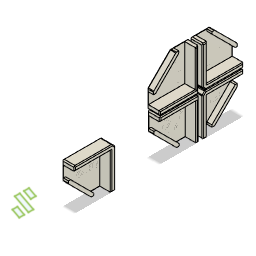
extrusion door corners v3 (Autodesk Fusion 360 design; units mm, degrees)
Autodesk Fusion 360 part; units mm, degrees
note: some values were not read from the file. Chosen so that the rebuilt part matches the saved one: which pieces of a blend or face edit are solid.
sketch "Sketch1" plane through (0, 0, 0) normal (0, 1, 0) x (1, 0, 0)
  line L0 (2, 2) -> (8, 2)
  line L1 (8, 2) -> (8, 8)
  line L2 (8, 8) -> (2, 8)
  line L3 (2, 8) -> (2, 2)
  line L4 (3.7738, 2) -> (6.1738, 2)
  line L5 (6.1738, 2) -> (6.1738, 6)
  line L6 (6.1738, 6) -> (3.7738, 6)
  line L7 (3.7738, 6) -> (3.7738, 2)
  dimension "d1" = 6
  dimension "d2" = 6
  dimension "d3" = 2.4
  dimension "d4" = 4
  constraint horizontal L0
  constraint vertical L1
  constraint horizontal L2
  constraint vertical L3
  constraint horizontal L4
  constraint vertical L5
  constraint horizontal L6
  constraint vertical L7
  constraint coincident L0 L4.start
  measures "d1" distance of L0.start L0.end
  measures "d2" distance of L0.start L2.end
  measures "d3" distance of L4.start L4.end
  measures "d4" distance of L4.start L6.end
sketch "Sketch2" plane through (0, 0, 0) normal (1, 0, 0) x (0, 0, -1)
  line L0 (-1.5, 1) -> (-73.5, 1)
  line L1 (-73.5, 1) -> (-73.5, 73)
  line L2 (-73.5, 73) -> (-1.5, 73)
  line L3 (-1.5, 73) -> (-1.5, 1)
  dimension "d20" = 72
  dimension "d21" = 72
  constraint horizontal L0
  constraint vertical L1
  constraint horizontal L2
  constraint vertical L3
  measures "d20" distance of L0.start L0.end
  measures "d21" distance of L0.start L2.end
extrude "Extrude2" add sketch "Sketch2" along normal blind 2 makes body 1
sketch "Sketch3" plane through (2, 0, 0) normal (1, 0, 0) x (0, 0, -1)
  line L0 (-1.5, 73) -> (-73.5, 73)
  line L1 (-73.5, 73) -> (-73.5, 1)
  line L2 (-73.5, 1) -> (-1.5, 1)
  line L3 (-1.5, 1) -> (-1.5, 73)
  line L4 (-1.5, 1) -> (-73.5, 1)
  line L5 (-73.5, 1) -> (-73.5, 8.8)
  line L6 (-73.5, 8.8) -> (-1.5, 8.8)
  line L7 (-1.5, 8.8) -> (-1.5, 1)
  line L8 (-1.5, 8.8) -> (-9.3, 8.8)
  line L9 (-9.3, 8.8) -> (-9.3, 73)
  line L10 (-9.3, 73) -> (-1.5, 73)
  line L11 (-1.5, 73) -> (-1.5, 8.8)
  dimension "d24" = 7.8
  dimension "d25" = 7.8
  constraint horizontal L4
  constraint vertical L5
  constraint horizontal L6
  constraint vertical L7
  constraint coincident L2.end L3.start
  constraint horizontal L8
  constraint vertical L9
  constraint horizontal L10
  constraint vertical L11
  measures "d24" distance of L2.end L6.end
  measures "d25" distance of L6.end L8.end
extrude "Extrude3" add sketch "Sketch3" along normal blind 20 contours L1 L2 L3 L4 L5 L6 L7 L8 bodies 1
sketch "Sketch4" plane through (2, 0, 0) normal (1, 0, 0) x (0, 0, -1)
  line L0 (-73.5, 8.8) -> (-1.5, 8.8)
  line L1 (-1.5, 8.8) -> (-1.5, 73)
  line L2 (-1.5, 73) -> (-73.5, 73)
  line L3 (-73.5, 73) -> (-73.5, 8.8)
  line L4 (-1.5, 8.8) -> (-9.3, 8.8)
  line L5 (-9.3, 8.8) -> (-9.3, 73)
  line L6 (-9.3, 73) -> (-1.5, 73)
  line L7 (-1.5, 73) -> (-1.5, 8.8)
  dimension "d28" = 7.8
  constraint horizontal L4
  constraint vertical L5
  constraint horizontal L6
  constraint vertical L7
  constraint coincident L0.end L1.start
  measures "d28" distance of L0.end L4.end
extrude "Extrude4" add sketch "Sketch4" along normal blind 7.8 contours L0 L1 L2 L4 L5 L6 L7 bodies 1
sketch "Sketch5" plane through (2, 0, 0) normal (1, 0, 0) x (0, 0, -1)
  line L0 (-9.3, 8.8) -> (-9.3, 73)
  line L1 (-9.3, 73) -> (-73.5, 73)
  line L2 (-73.5, 73) -> (-73.5, 8.8)
  line L3 (-73.5, 8.8) -> (-9.3, 8.8)
  line L4 (-73.5, 73) -> (-28.828, 73)
  line L5 (-28.828, 73) -> (-28.828, 28.328)
  line L6 (-28.828, 28.328) -> (-73.5, 28.328)
  line L7 (-73.5, 28.328) -> (-73.5, 73)
  dimension "d31" = 44.672
  dimension "d32" = 44.672
  constraint horizontal L4
  constraint vertical L5
  constraint horizontal L6
  constraint vertical L7
  constraint coincident L1.end L2.start
  measures "d31" distance of L1.end L4.end
  measures "d32" distance of L1.end L6.end
extrude "Extrude5" add sketch "Sketch5" along normal blind 9 contours L1 L2 L4 L5 L6 L7 bodies 1
extrude "Extrude6" add 1 faces at (9.8, 51.6, 6.7) along direction (1, 0, 0) blind 12 on bodies 1 bodies 1
extrude "Extrude7" add 1 faces at (21.8, 51.6, 6.7) along direction (1, 0, 0) blind 0.2 on bodies 1 bodies 1
chamfer "Chamfer6" distance 40 angle 45 1 edges at (5.5, 73, 73.5) on bodies 1
chamfer "Chamfer9" distance 41 angle 45 1 edges at (6.5, 28.328, 28.828) on bodies 1
chamfer "Chamfer12" distance 1.5 angle 45 1 faces at (0, 35.6667, 36.1667) on bodies 1
chamfer "Chamfer13" distance 1.5 angle 45 1 faces at (22, 3.6, 28.1) on bodies 1
fillet "Fillet4" radius 2 4 edges at (11, 1, 73.5) (6.25, 73, 33.5) (6.25, 33, 73.5) (11, 73, 1.5) on bodies 1
chamfer "Chamfer14" distance 5 angle 45 1 edges at (11, 1, 1.5) on bodies 1
chamfer "Chamfer15" distance 1.5 angle 45 2 edges at (0, 3.5, 4) (22, 3.5, 4) on bodies 1
fillet "Fillet5" radius 2 2 edges at (11, 1, 6.5) (11, 6, 1.5) on bodies 1
sketch "Sketch6" plane through (0, 0, 0) normal (1, 0, 0) x (0, 0, -1)
  line L0 (37.7693, -15.5046) -> (28.9904, -15.5046)
  line L1 (28.9904, -15.5046) -> (40.9998, -33.7714)
  line L2 (40.9998, -33.7714) -> (49.7787, -33.7714)
  line L3 (49.7787, -33.7714) -> (37.7693, -15.5046)
  line L4 (45.6089, -52.0171) -> (21.5926, -15.4781)
  line L5 (21.5926, -15.4781) -> (12.8138, -15.4781)
  line L6 (12.8138, -15.4781) -> (36.8327, -52.0171)
  line L7 (36.8327, -52.0171) -> (45.6089, -52.0171)
  line L8 (20.6507, -52.0171) -> (29.4296, -52.0171)
  line L9 (29.4296, -52.0171) -> (17.4228, -33.7503)
  line L10 (17.4228, -33.7503) -> (8.6439, -33.7503)
  line L11 (8.6439, -33.7503) -> (20.6507, -52.0171)
copy_body "CopyPasteBodies1" bodies 1 makes body 2
move_body "Move1" bodies 2 to x (1, 0, 0) y (0, 1, 0) z (0, 0, 1) at (0, 0, 155)
mirror "Mirror1" about plane through (0, 0, 0) normal (0, 0, 1) of bodies 2 makes body 3
mirror "Mirror2" about plane through (0, 0, 0) normal (0, 1, 0) of bodies 3 makes body 4
mirror "Mirror3" about plane through (0, 0, 0) normal (0, 1, 0) of bodies 1 makes body 5
move_body "Move2" bodies 1 to x (1, 0, 0) y (0, 1, 0) z (0, 0, 1) at (0, 0, -320)
move_body "Move3" bodies 4 to x (1, 0, 0) y (0, 1, 0) z (0, 0, 1) at (0, 150, 0)
move_body "Move4" bodies 5 to x (1, 0, 0) y (0, 1, 0) z (0, 0, 1) at (0, 150, -320)
sketch "Sketch7" plane through (0, 0, 0) normal (-1, 0, 0) x (0, 0, 1)
  line L0 (-162.1213, 2.5) -> (-158, 6.6213)
  line L1 (-158, 6.6213) -> (-158, 71.5)
  line L2 (-158, 71.5) -> (-187.8787, 71.5)
  line L3 (-187.8787, 71.5) -> (-227, 32.3787)
  line L4 (-227, 32.3787) -> (-227, 2.5)
  line L5 (-227, 2.5) -> (-162.1213, 2.5)
  line L6 (-196.3905, 49.0459) -> (-188.4895, 49.0459)
  line L7 (-188.4895, 49.0459) -> (-199.298, 32.6057)
  line L8 (-199.298, 32.6057) -> (-207.199, 32.6057)
  line L9 (-207.199, 32.6057) -> (-196.3905, 49.0459)
  line L10 (-203.4462, 16.1846) -> (-181.8316, 49.0697)
  line L11 (-181.8316, 49.0697) -> (-173.9306, 49.0697)
  line L12 (-173.9306, 49.0697) -> (-195.5476, 16.1846)
  line L13 (-195.5476, 16.1846) -> (-203.4462, 16.1846)
  line L14 (-180.9838, 16.1846) -> (-188.8848, 16.1846)
  line L15 (-188.8848, 16.1846) -> (-178.0787, 32.6248)
  line L16 (-178.0787, 32.6248) -> (-170.1777, 32.6248)
  line L17 (-170.1777, 32.6248) -> (-180.9838, 16.1846)
extrude "Extrude8" cut sketch "Sketch7" against normal blind 0.7 contours L6 L7 L8 L9 | L10 L11 L12 L13 | L14 L15 L16 L17 bodies 3
sketch "Sketch8" plane through (0, 0, 0) normal (-1, 0, 0) x (0, 0, 1)
  line L0 (-317, 6.6213) -> (-312.8787, 2.5)
  line L1 (-312.8787, 2.5) -> (-248, 2.5)
  line L2 (-248, 2.5) -> (-248, 32.3787)
  line L3 (-248, 32.3787) -> (-287.1213, 71.5)
  line L4 (-287.1213, 71.5) -> (-317, 71.5)
  line L5 (-317, 71.5) -> (-317, 6.6213)
  line L6 (-296.3905, 49.0459) -> (-288.4895, 49.0459)
  line L7 (-288.4895, 49.0459) -> (-299.298, 32.6057)
  line L8 (-299.298, 32.6057) -> (-307.199, 32.6057)
  line L9 (-307.199, 32.6057) -> (-296.3905, 49.0459)
  line L10 (-303.4462, 16.1846) -> (-281.8316, 49.0697)
  line L11 (-281.8316, 49.0697) -> (-273.9306, 49.0697)
  line L12 (-273.9306, 49.0697) -> (-295.5476, 16.1846)
  line L13 (-295.5476, 16.1846) -> (-303.4462, 16.1846)
  line L14 (-280.9838, 16.1846) -> (-288.8848, 16.1846)
  line L15 (-288.8848, 16.1846) -> (-278.0787, 32.6248)
  line L16 (-278.0787, 32.6248) -> (-270.1777, 32.6248)
  line L17 (-270.1777, 32.6248) -> (-280.9838, 16.1846)
extrude "Extrude9" cut sketch "Sketch8" against normal blind 0.7 contours L6 L7 L8 L9 | L10 L11 L12 L13 | L14 L15 L16 L17 bodies 1
sketch "Sketch9" plane through (0, 0, 0) normal (-1, 0, 0) x (0, 0, 1)
  line L0 (-158, 143.3787) -> (-162.1213, 147.5)
  line L1 (-162.1213, 147.5) -> (-227, 147.5)
  line L2 (-227, 147.5) -> (-227, 117.6213)
  line L3 (-227, 117.6213) -> (-187.8787, 78.5)
  line L4 (-187.8787, 78.5) -> (-158, 78.5)
  line L5 (-158, 78.5) -> (-158, 143.3787)
  line L6 (-164.2409, 106.1512) -> (-169.8403, 106.1512)
  line L7 (-169.8403, 106.1512) -> (-176.0067, 124.5441)
  line L8 (-176.0067, 124.5441) -> (-176.1485, 124.5441)
  line L9 (-176.1485, 124.5441) -> (-182.3149, 106.1512)
  line L10 (-182.3149, 106.1512) -> (-187.7725, 106.1512)
  line L11 (-187.7725, 106.1512) -> (-179.2671, 129.1512)
  line L12 (-179.2671, 129.1512) -> (-172.4983, 129.1512)
  line L13 (-172.4983, 129.1512) -> (-164.2409, 106.1512)
  spline S0 degree 2 poles (-189.828, 123.9062) (-189.828, 121.9925) (-190.8912, 120.5749) knots 0 0 0 1 1 1
  spline S1 degree 2 poles (-190.8912, 120.5749) (-191.9544, 119.1573) (-193.6554, 118.4131) knots 0 0 0 1 1 1
  spline S2 degree 2 poles (-193.6554, 118.4131) (-195.0021, 117.8107) (-196.8095, 117.2082) knots 0 0 0 1 1 1
  spline S3 degree 2 poles (-196.8095, 117.2082) (-198.6169, 116.6057) (-199.6092, 115.9324) knots 0 0 0 1 1 1
  spline S4 degree 2 poles (-199.6092, 115.9324) (-200.6015, 115.259) (-200.6015, 114.3376) knots 0 0 0 1 1 1
  line L14 (-200.6015, 114.3376) -> (-200.6015, 111.3962)
  spline S5 degree 2 poles (-200.6015, 111.3962) (-200.6015, 110.2976) (-199.7155, 109.9432) knots 0 0 0 1 1 1
  spline S6 degree 2 poles (-199.7155, 109.9432) (-198.7587, 109.5533) (-196.7386, 109.5533) knots 0 0 0 1 1 1
  spline S7 degree 2 poles (-196.7386, 109.5533) (-194.2933, 109.5533) (-190.2887, 110.4393) knots 0 0 0 1 1 1
  line L15 (-190.2887, 110.4393) -> (-190.2887, 106.541)
  spline S8 degree 2 poles (-190.2887, 106.541) (-193.8326, 105.7968) (-197.6955, 105.7968) knots 0 0 0 1 1 1
  spline S9 degree 2 poles (-197.6955, 105.7968) (-201.8773, 105.7968) (-203.9151, 107.0726) knots 0 0 0 1 1 1
  spline S10 degree 2 poles (-203.9151, 107.0726) (-205.9528, 108.3484) (-205.9528, 111.3253) knots 0 0 0 1 1 1
  line L16 (-205.9528, 111.3253) -> (-205.9528, 114.5148)
  spline S11 degree 2 poles (-205.9528, 114.5148) (-205.9528, 116.3222) (-204.8719, 117.6512) knots 0 0 0 1 1 1
  spline S12 degree 2 poles (-204.8719, 117.6512) (-203.791, 118.9801) (-202.0899, 119.6535) knots 0 0 0 1 1 1
  spline S13 degree 2 poles (-202.0899, 119.6535) (-200.4952, 120.3268) (-198.8295, 120.8584) knots 0 0 0 1 1 1
  spline S14 degree 2 poles (-198.8295, 120.8584) (-197.0222, 121.4963) (-195.9767, 122.276) knots 0 0 0 1 1 1
  spline S15 degree 2 poles (-195.9767, 122.276) (-194.9312, 123.0556) (-194.9312, 124.1188) knots 0 0 0 1 1 1
  line L17 (-194.9312, 124.1188) -> (-194.9312, 125.2883)
  line L18 (-194.9312, 125.2883) -> (-205.9883, 125.2883)
  line L19 (-205.9883, 125.2883) -> (-205.9883, 129.1512)
  line L20 (-205.9883, 129.1512) -> (-189.828, 129.1512)
  line L21 (-189.828, 129.1512) -> (-189.828, 123.9062)
extrude "Extrude10" cut sketch "Sketch9" against normal blind 0.7 contours L6 L7 L8 L9 L10 L11 L12 L13 | S0 S1 S2 S3 S4 L14 S5 S6 S7 L15 S8 S9 S10 L16 S11 S12 S13 S14 S15 L17 L18 L19 L20 L21 bodies 4
sketch "Sketch10" plane through (0, 0, 0) normal (-1, 0, 0) x (0, 0, 1)
  line L0 (-312.8787, 147.5) -> (-317, 143.3787)
  line L1 (-317, 143.3787) -> (-317, 78.5)
  line L2 (-317, 78.5) -> (-287.1213, 78.5)
  line L3 (-287.1213, 78.5) -> (-248, 117.6213)
  line L4 (-248, 117.6213) -> (-248, 147.5)
  line L5 (-248, 147.5) -> (-312.8787, 147.5)
  line L6 (-168.6342, 139.35) -> (-167.4416, 139.35)
  line L7 (-167.4416, 139.35) -> (-167.4416, 138.2544)
  line L8 (-167.4416, 138.2544) -> (-168.8561, 138.2544)
  line L9 (-168.8561, 138.2544) -> (-169.1612, 136.8122)
  line L10 (-169.1612, 136.8122) -> (-167.4416, 136.8122)
  line L11 (-167.4416, 136.8122) -> (-167.4416, 135.7028)
  line L12 (-167.4416, 135.7028) -> (-169.3831, 135.7028)
  line L13 (-169.3831, 135.7028) -> (-169.8962, 133.1651)
  line L14 (-169.8962, 133.1651) -> (-171.0888, 133.1651)
  line L15 (-171.0888, 133.1651) -> (-170.5757, 135.7028)
  line L16 (-170.5757, 135.7028) -> (-171.4632, 135.7028)
  line L17 (-171.4632, 135.7028) -> (-171.9763, 133.1651)
  line L18 (-171.9763, 133.1651) -> (-173.1689, 133.1651)
  line L19 (-173.1689, 133.1651) -> (-172.6558, 135.7028)
  line L20 (-172.6558, 135.7028) -> (-173.8207, 135.7028)
  line L21 (-173.8207, 135.7028) -> (-173.8207, 136.8122)
  line L22 (-173.8207, 136.8122) -> (-172.4201, 136.8122)
  line L23 (-172.4201, 136.8122) -> (-172.1288, 138.2544)
  line L24 (-172.1288, 138.2544) -> (-173.8207, 138.2544)
  line L25 (-173.8207, 138.2544) -> (-173.8207, 139.35)
  line L26 (-173.8207, 139.35) -> (-171.907, 139.35)
  line L27 (-171.907, 139.35) -> (-171.3661, 142.0264)
  line L28 (-171.3661, 142.0264) -> (-170.1735, 142.0264)
  line L29 (-170.1735, 142.0264) -> (-170.7144, 139.35)
  line L30 (-170.7144, 139.35) -> (-169.8268, 139.35)
  line L31 (-169.8268, 139.35) -> (-169.286, 142.0264)
  line L32 (-169.286, 142.0264) -> (-168.0934, 142.0264)
  line L33 (-168.0934, 142.0264) -> (-168.6342, 139.35)
  line L34 (-170.9362, 138.2544) -> (-171.2413, 136.8122)
  line L35 (-171.2413, 136.8122) -> (-170.3399, 136.8122)
  line L36 (-170.3399, 136.8122) -> (-170.0487, 138.2544)
  line L37 (-170.0487, 138.2544) -> (-170.9362, 138.2544)
  line L38 (-178.286, 135.1481) -> (-175.8315, 136.5071)
  line L39 (-175.8315, 136.5071) -> (-175.8315, 134.8014)
  line L40 (-175.8315, 134.8014) -> (-178.6743, 133.0264)
  line L41 (-178.6743, 133.0264) -> (-180.3107, 133.0264)
  line L42 (-180.3107, 133.0264) -> (-180.3107, 142.0264)
  line L43 (-180.3107, 142.0264) -> (-178.286, 142.0264)
  line L44 (-178.286, 142.0264) -> (-178.286, 135.1481)
  line L45 (-186.3291, 135.1481) -> (-183.8746, 136.5071)
  line L46 (-183.8746, 136.5071) -> (-183.8746, 134.8014)
  line L47 (-183.8746, 134.8014) -> (-186.7174, 133.0264)
  line L48 (-186.7174, 133.0264) -> (-188.3538, 133.0264)
  line L49 (-188.3538, 133.0264) -> (-188.3538, 142.0264)
  line L50 (-188.3538, 142.0264) -> (-186.3291, 142.0264)
  line L51 (-186.3291, 142.0264) -> (-186.3291, 135.1481)
  line L52 (-195.2598, 140.2097) -> (-191.0996, 140.2097)
  line L53 (-191.0996, 140.2097) -> (-191.0996, 138.615)
  line L54 (-191.0996, 138.615) -> (-194.8022, 133.0264)
  line L55 (-194.8022, 133.0264) -> (-197.0903, 133.0264)
  line L56 (-197.0903, 133.0264) -> (-197.0903, 138.7537)
  line L57 (-197.0903, 138.7537) -> (-198.061, 138.7537)
  line L58 (-198.061, 138.7537) -> (-198.061, 140.2097)
  line L59 (-198.061, 140.2097) -> (-197.0903, 140.2097)
  line L60 (-197.0903, 140.2097) -> (-197.0903, 142.0264)
  line L61 (-197.0903, 142.0264) -> (-195.2598, 142.0264)
  line L62 (-195.2598, 142.0264) -> (-195.2598, 140.2097)
  line L63 (-195.2598, 138.7537) -> (-195.2598, 134.9401)
  line L64 (-195.2598, 134.9401) -> (-192.833, 138.7537)
  line L65 (-192.833, 138.7537) -> (-195.2598, 138.7537)
  spline S0 degree 2 poles (-202.457, 142.1651) (-201.2922, 142.1651) (-199.4339, 141.957) knots 0 0 0 1 1 1
  line L66 (-199.4339, 141.957) -> (-199.4339, 140.3484)
  line L67 (-199.4339, 140.3484) -> (-199.8777, 140.4316)
  spline S1 degree 2 poles (-199.8777, 140.4316) (-200.1412, 140.4871) (-200.1689, 140.501) knots 0 0 0 1 1 1
  line L68 (-200.1689, 140.501) -> (-200.6404, 140.5842)
  spline S2 degree 2 poles (-200.6404, 140.5842) (-200.8068, 140.6119) (-201.3476, 140.6674) knots 0 0 0 1 1 1
  spline S3 degree 2 poles (-201.3476, 140.6674) (-201.7637, 140.709) (-202.1936, 140.709) knots 0 0 0 1 1 1
  spline S4 degree 2 poles (-202.1936, 140.709) (-202.9979, 140.709) (-203.3099, 140.5148) knots 0 0 0 1 1 1
  spline S5 degree 2 poles (-203.3099, 140.5148) (-203.6219, 140.3207) (-203.6219, 139.7799) knots 0 0 0 1 1 1
  line L69 (-203.6219, 139.7799) -> (-203.6219, 138.7398)
  spline S6 degree 2 poles (-203.6219, 138.7398) (-203.6219, 138.088) (-202.2213, 138.088) knots 0 0 0 1 1 1
  line L70 (-202.2213, 138.088) -> (-200.5849, 138.088)
  line L71 (-200.5849, 138.088) -> (-200.5849, 136.7013)
  line L72 (-200.5849, 136.7013) -> (-202.2213, 136.7013)
  spline S7 degree 2 poles (-202.2213, 136.7013) (-203.303, 136.7013) (-203.303, 135.9108) knots 0 0 0 1 1 1
  line L73 (-203.303, 135.9108) -> (-203.303, 135.0372)
  spline S8 degree 2 poles (-203.303, 135.0372) (-203.303, 134.746) (-203.192, 134.5865) knots 0 0 0 1 1 1
  spline S9 degree 2 poles (-203.192, 134.5865) (-203.0811, 134.427) (-202.7968, 134.3577) knots 0 0 0 1 1 1
  spline S10 degree 2 poles (-202.7968, 134.3577) (-202.5125, 134.2883) (-201.9578, 134.2883) knots 0 0 0 1 1 1
  spline S11 degree 2 poles (-201.9578, 134.2883) (-201.1674, 134.2883) (-199.5171, 134.4547) knots 0 0 0 1 1 1
  line L74 (-199.5171, 134.4547) -> (-199.5171, 133.0125)
  spline S12 degree 2 poles (-199.5171, 133.0125) (-201.4031, 132.8877) (-202.1797, 132.8877) knots 0 0 0 1 1 1
  spline S13 degree 2 poles (-202.1797, 132.8877) (-203.8715, 132.8877) (-204.6273, 133.276) knots 0 0 0 1 1 1
  spline S14 degree 2 poles (-204.6273, 133.276) (-205.3831, 133.6643) (-205.3831, 134.6489) knots 0 0 0 1 1 1
  line L75 (-205.3831, 134.6489) -> (-205.3831, 136.1327)
  spline S15 degree 2 poles (-205.3831, 136.1327) (-205.3831, 136.5349) (-205.1404, 136.8191) knots 0 0 0 1 1 1
  spline S16 degree 2 poles (-205.1404, 136.8191) (-204.8977, 137.1034) (-204.5233, 137.2005) knots 0 0 0 1 1 1
  spline S17 degree 2 poles (-204.5233, 137.2005) (-205.7436, 137.6304) (-205.7436, 138.5456) knots 0 0 0 1 1 1
  line L76 (-205.7436, 138.5456) -> (-205.7436, 140.0156)
  spline S18 degree 2 poles (-205.7436, 140.0156) (-205.7436, 141.1666) (-204.9532, 141.6658) knots 0 0 0 1 1 1
  spline S19 degree 2 poles (-204.9532, 141.6658) (-204.1627, 142.1651) (-202.457, 142.1651) knots 0 0 0 1 1 1
  line L77 (-267.4991, 108.339) -> (-269.9028, 108.339)
  line L78 (-269.9028, 108.339) -> (-269.9028, 118.339)
  line L79 (-269.9028, 118.339) -> (-267.4991, 118.339)
  line L80 (-267.4991, 118.339) -> (-267.4991, 108.339)
  line L81 (-269.9644, 113.0385) -> (-273.7087, 108.339)
  line L82 (-273.7087, 108.339) -> (-276.5284, 108.339)
  line L83 (-276.5284, 108.339) -> (-272.7379, 112.9923)
  line L84 (-272.7379, 112.9923) -> (-276.9444, 118.339)
  line L85 (-276.9444, 118.339) -> (-274.0168, 118.339)
  line L86 (-274.0168, 118.339) -> (-269.9644, 113.0385)
  line L87 (-280.6732, 114.3328) -> (-277.0523, 108.339)
  line L88 (-277.0523, 108.339) -> (-279.7795, 108.339)
  line L89 (-279.7795, 108.339) -> (-281.8905, 112.2527)
  line L90 (-281.8905, 112.2527) -> (-283.986, 108.339)
  line L91 (-283.986, 108.339) -> (-286.7287, 108.339)
  line L92 (-286.7287, 108.339) -> (-283.0769, 114.302)
  line L93 (-283.0769, 114.302) -> (-283.0769, 118.339)
  line L94 (-283.0769, 118.339) -> (-280.6732, 118.339)
  line L95 (-280.6732, 118.339) -> (-280.6732, 114.3328)
  line L96 (-287.9305, 108.339) -> (-292.4298, 108.339)
  spline S20 degree 2 poles (-292.4298, 108.339) (-294.4329, 108.339) (-295.3265, 108.8243) knots 0 0 0 1 1 1
  spline S21 degree 2 poles (-295.3265, 108.8243) (-296.2202, 109.3097) (-296.2202, 110.4499) knots 0 0 0 1 1 1
  line L97 (-296.2202, 110.4499) -> (-296.2202, 112.2065)
  spline S22 degree 2 poles (-296.2202, 112.2065) (-296.2202, 113.0847) (-295.5962, 113.5855) knots 0 0 0 1 1 1
  spline S23 degree 2 poles (-295.5962, 113.5855) (-294.9721, 114.0863) (-293.9398, 114.225) knots 0 0 0 1 1 1
  line L98 (-293.9398, 114.225) -> (-296.8366, 118.339)
  line L99 (-296.8366, 118.339) -> (-294.0631, 118.339)
  line L100 (-294.0631, 118.339) -> (-291.4436, 114.4099)
  line L101 (-291.4436, 114.4099) -> (-290.3342, 114.4099)
  line L102 (-290.3342, 114.4099) -> (-290.3342, 118.339)
  line L103 (-290.3342, 118.339) -> (-287.9305, 118.339)
  line L104 (-287.9305, 118.339) -> (-287.9305, 108.339)
  spline S24 degree 2 poles (-292.399, 112.8228) (-293.2464, 112.8228) (-293.5546, 112.5994) knots 0 0 0 1 1 1
  spline S25 degree 2 poles (-293.5546, 112.5994) (-293.8627, 112.376) (-293.8627, 111.7288) knots 0 0 0 1 1 1
  line L105 (-293.8627, 111.7288) -> (-293.8627, 111.02)
  spline S26 degree 2 poles (-293.8627, 111.02) (-293.8627, 110.4653) (-293.5315, 110.2573) knots 0 0 0 1 1 1
  spline S27 degree 2 poles (-293.5315, 110.2573) (-293.2002, 110.0493) (-292.399, 110.0493) knots 0 0 0 1 1 1
  line L106 (-292.399, 110.0493) -> (-290.3342, 110.0493)
  line L107 (-290.3342, 110.0493) -> (-290.3342, 112.8228)
  line L108 (-290.3342, 112.8228) -> (-292.399, 112.8228)
  spline S28 degree 2 poles (-302.7379, 118.4931) (-301.9059, 118.4931) (-301.2048, 118.3852) knots 0 0 0 1 1 1
  spline S29 degree 2 poles (-301.2048, 118.3852) (-300.5037, 118.2774) (-299.7487, 118.0154) knots 0 0 0 1 1 1
  spline S30 degree 2 poles (-299.7487, 118.0154) (-298.9321, 117.7381) (-298.4698, 117.114) knots 0 0 0 1 1 1
  spline S31 degree 2 poles (-298.4698, 117.114) (-298.0076, 116.49) (-298.0076, 115.5963) knots 0 0 0 1 1 1
  line L109 (-298.0076, 115.5963) -> (-298.0076, 111.2203)
  spline S32 degree 2 poles (-298.0076, 111.2203) (-298.0076, 110.4807) (-298.3389, 109.8952) knots 0 0 0 1 1 1
  spline S33 degree 2 poles (-298.3389, 109.8952) (-298.6701, 109.3097) (-299.194, 108.9707) knots 0 0 0 1 1 1
  spline S34 degree 2 poles (-299.194, 108.9707) (-299.6563, 108.678) (-300.3342, 108.4777) knots 0 0 0 1 1 1
  spline S35 degree 2 poles (-300.3342, 108.4777) (-301.0122, 108.2774) (-301.5977, 108.2311) knots 0 0 0 1 1 1
  spline S36 degree 2 poles (-301.5977, 108.2311) (-302.137, 108.1849) (-302.7379, 108.1849) knots 0 0 0 1 1 1
  spline S37 degree 2 poles (-302.7379, 108.1849) (-303.4467, 108.1849) (-303.9706, 108.2388) knots 0 0 0 1 1 1
  spline S38 degree 2 poles (-303.9706, 108.2388) (-304.4945, 108.2928) (-305.1416, 108.4623) knots 0 0 0 1 1 1
  spline S39 degree 2 poles (-305.1416, 108.4623) (-305.8812, 108.678) (-306.3589, 108.9861) knots 0 0 0 1 1 1
  spline S40 degree 2 poles (-306.3589, 108.9861) (-306.8366, 109.2943) (-307.1601, 109.849) knots 0 0 0 1 1 1
  spline S41 degree 2 poles (-307.1601, 109.849) (-307.4991, 110.4191) (-307.4991, 111.2203) knots 0 0 0 1 1 1
  line L110 (-307.4991, 111.2203) -> (-307.4991, 115.5963)
  spline S42 degree 2 poles (-307.4991, 115.5963) (-307.4991, 116.4284) (-307.06, 117.0293) knots 0 0 0 1 1 1
  spline S43 degree 2 poles (-307.06, 117.0293) (-306.6208, 117.6302) (-305.8504, 117.9384) knots 0 0 0 1 1 1
  spline S44 degree 2 poles (-305.8504, 117.9384) (-304.4637, 118.4931) (-302.7379, 118.4931) knots 0 0 0 1 1 1
  spline S45 degree 2 poles (-302.7688, 116.7827) (-303.2772, 116.7827) (-303.6239, 116.7442) knots 0 0 0 1 1 1
  spline S46 degree 2 poles (-303.6239, 116.7442) (-303.9706, 116.7057) (-304.3404, 116.5978) knots 0 0 0 1 1 1
  spline S47 degree 2 poles (-304.3404, 116.5978) (-304.7102, 116.49) (-304.9028, 116.2357) knots 0 0 0 1 1 1
  spline S48 degree 2 poles (-304.9028, 116.2357) (-305.0954, 115.9815) (-305.0954, 115.5963) knots 0 0 0 1 1 1
  line L111 (-305.0954, 115.5963) -> (-305.0954, 111.2049)
  spline S49 degree 2 poles (-305.0954, 111.2049) (-305.0954, 110.4962) (-304.5253, 110.1957) knots 0 0 0 1 1 1
  spline S50 degree 2 poles (-304.5253, 110.1957) (-303.9552, 109.8952) (-302.7533, 109.8952) knots 0 0 0 1 1 1
  spline S51 degree 2 poles (-302.7533, 109.8952) (-301.5515, 109.8952) (-300.9814, 110.188) knots 0 0 0 1 1 1
  spline S52 degree 2 poles (-300.9814, 110.188) (-300.4113, 110.4807) (-300.4113, 111.2049) knots 0 0 0 1 1 1
  line L112 (-300.4113, 111.2049) -> (-300.4113, 115.5963)
  spline S53 degree 2 poles (-300.4113, 115.5963) (-300.4113, 115.9815) (-300.6116, 116.2357) knots 0 0 0 1 1 1
  spline S54 degree 2 poles (-300.6116, 116.2357) (-300.8119, 116.49) (-301.1971, 116.5978) knots 0 0 0 1 1 1
  spline S55 degree 2 poles (-301.1971, 116.5978) (-301.5669, 116.7057) (-301.9136, 116.7442) knots 0 0 0 1 1 1
  spline S56 degree 2 poles (-301.9136, 116.7442) (-302.2603, 116.7827) (-302.7688, 116.7827) knots 0 0 0 1 1 1
  line L113 (-269.2942, 128) -> (-271.6979, 128)
  line L114 (-271.6979, 128) -> (-271.6979, 136.2897)
  line L115 (-271.6979, 136.2897) -> (-276.6131, 136.2897)
  line L116 (-276.6131, 136.2897) -> (-276.6131, 138)
  line L117 (-276.6131, 138) -> (-269.2942, 138)
  line L118 (-269.2942, 138) -> (-269.2942, 128)
  line L119 (-280.8812, 128) -> (-283.8088, 128)
  line L120 (-283.8088, 128) -> (-287.4144, 138)
  line L121 (-287.4144, 138) -> (-284.9799, 138)
  line L122 (-284.9799, 138) -> (-284.0862, 135.3652)
  line L123 (-284.0862, 135.3652) -> (-280.4344, 135.3652)
  line L124 (-280.4344, 135.3652) -> (-279.5561, 138)
  line L125 (-279.5561, 138) -> (-277.1832, 138)
  line L126 (-277.1832, 138) -> (-280.8812, 128)
  line L127 (-283.5623, 133.7627) -> (-282.2988, 130.0031)
  line L128 (-282.2988, 130.0031) -> (-282.2372, 130.0031)
  line L129 (-282.2372, 130.0031) -> (-280.9737, 133.7627)
  line L130 (-280.9737, 133.7627) -> (-283.5623, 133.7627)
  line L131 (-288.5238, 128) -> (-292.5762, 128)
  spline S57 degree 2 poles (-292.5762, 128) (-294.0091, 128) (-294.7872, 128.208) knots 0 0 0 1 1 1
  spline S58 degree 2 poles (-294.7872, 128.208) (-295.5654, 128.416) (-295.8889, 128.8706) knots 0 0 0 1 1 1
  spline S59 degree 2 poles (-295.8889, 128.8706) (-296.2125, 129.3251) (-296.2125, 130.1418) knots 0 0 0 1 1 1
  line L132 (-296.2125, 130.1418) -> (-296.2125, 131.3744)
  spline S60 degree 2 poles (-296.2125, 131.3744) (-296.2125, 131.7904) (-295.8812, 132.1602) knots 0 0 0 1 1 1
  spline S61 degree 2 poles (-295.8812, 132.1602) (-295.55, 132.53) (-295.1031, 132.6687) knots 0 0 0 1 1 1
  line L133 (-295.1031, 132.6687) -> (-295.1031, 132.7458)
  spline S62 degree 2 poles (-295.1031, 132.7458) (-295.6886, 132.8074) (-296.174, 133.2465) knots 0 0 0 1 1 1
  spline S63 degree 2 poles (-296.174, 133.2465) (-296.6594, 133.6857) (-296.6594, 134.225) knots 0 0 0 1 1 1
  line L134 (-296.6594, 134.225) -> (-296.6594, 135.7658)
  spline S64 degree 2 poles (-296.6594, 135.7658) (-296.6594, 136.983) (-295.6886, 137.4915) knots 0 0 0 1 1 1
  spline S65 degree 2 poles (-295.6886, 137.4915) (-294.7179, 138) (-292.684, 138) knots 0 0 0 1 1 1
  line L135 (-292.684, 138) -> (-288.5238, 138)
  line L136 (-288.5238, 138) -> (-288.5238, 128)
  spline S66 degree 2 poles (-292.5762, 132.0678) (-293.1463, 132.0678) (-293.4236, 131.9753) knots 0 0 0 1 1 1
  spline S67 degree 2 poles (-293.4236, 131.9753) (-293.701, 131.8829) (-293.8011, 131.6749) knots 0 0 0 1 1 1
  spline S68 degree 2 poles (-293.8011, 131.6749) (-293.9013, 131.4669) (-293.9013, 131.0663) knots 0 0 0 1 1 1
  line L137 (-293.9013, 131.0663) -> (-293.9013, 130.5732)
  spline S69 degree 2 poles (-293.9013, 130.5732) (-293.9013, 130.2188) (-293.8088, 130.0416) knots 0 0 0 1 1 1
  spline S70 degree 2 poles (-293.8088, 130.0416) (-293.7164, 129.8644) (-293.4313, 129.7874) knots 0 0 0 1 1 1
  spline S71 degree 2 poles (-293.4313, 129.7874) (-293.1463, 129.7103) (-292.5299, 129.7103) knots 0 0 0 1 1 1
  line L138 (-292.5299, 129.7103) -> (-290.9275, 129.7103)
  line L139 (-290.9275, 129.7103) -> (-290.9275, 132.0678)
  line L140 (-290.9275, 132.0678) -> (-292.5762, 132.0678)
  spline S72 degree 2 poles (-292.6378, 136.2897) (-293.5161, 136.2897) (-293.8859, 136.0894) knots 0 0 0 1 1 1
  spline S73 degree 2 poles (-293.8859, 136.0894) (-294.2557, 135.8891) (-294.2557, 135.4422) knots 0 0 0 1 1 1
  line L141 (-294.2557, 135.4422) -> (-294.2557, 134.641)
  spline S74 degree 2 poles (-294.2557, 134.641) (-294.2557, 134.0863) (-293.9706, 133.8552) knots 0 0 0 1 1 1
  spline S75 degree 2 poles (-293.9706, 133.8552) (-293.6856, 133.624) (-292.9614, 133.624) knots 0 0 0 1 1 1
  line L142 (-292.9614, 133.624) -> (-290.9275, 133.624)
  line L143 (-290.9275, 133.624) -> (-290.9275, 136.2897)
  line L144 (-290.9275, 136.2897) -> (-292.6378, 136.2897)
  spline S76 degree 2 poles (-301.5438, 138.1541) (-300.1108, 138.1541) (-297.9999, 137.8767) knots 0 0 0 1 1 1
  line L145 (-297.9999, 137.8767) -> (-297.9999, 136.0431)
  spline S77 degree 2 poles (-297.9999, 136.0431) (-300.6193, 136.4438) (-301.5746, 136.4438) knots 0 0 0 1 1 1
  spline S78 degree 2 poles (-301.5746, 136.4438) (-303.5777, 136.4438) (-303.5777, 135.4114) knots 0 0 0 1 1 1
  line L146 (-303.5777, 135.4114) -> (-303.5777, 134.7643)
  spline S79 degree 2 poles (-303.5777, 134.7643) (-303.5777, 134.2712) (-303.2926, 134.0092) knots 0 0 0 1 1 1
  spline S80 degree 2 poles (-303.2926, 134.0092) (-303.0076, 133.7473) (-302.268, 133.7473) knots 0 0 0 1 1 1
  line L147 (-302.268, 133.7473) -> (-301.097, 133.7473)
  spline S81 degree 2 poles (-301.097, 133.7473) (-297.7996, 133.7473) (-297.7996, 131.1279) knots 0 0 0 1 1 1
  line L148 (-297.7996, 131.1279) -> (-297.7996, 130.3883)
  spline S82 degree 2 poles (-297.7996, 130.3883) (-297.7996, 129.0786) (-298.8936, 128.4623) knots 0 0 0 1 1 1
  spline S83 degree 2 poles (-298.8936, 128.4623) (-299.9876, 127.8459) (-302.3604, 127.8459) knots 0 0 0 1 1 1
  spline S84 degree 2 poles (-302.3604, 127.8459) (-303.5931, 127.8459) (-305.4883, 128.0462) knots 0 0 0 1 1 1
  line L149 (-305.4883, 128.0462) -> (-305.4883, 129.8336)
  spline S85 degree 2 poles (-305.4883, 129.8336) (-303.1617, 129.5562) (-302.2834, 129.5562) knots 0 0 0 1 1 1
  spline S86 degree 2 poles (-302.2834, 129.5562) (-301.0661, 129.5562) (-300.6501, 129.7565) knots 0 0 0 1 1 1
  spline S87 degree 2 poles (-300.6501, 129.7565) (-300.2033, 129.9723) (-300.2033, 130.4345) knots 0 0 0 1 1 1
  line L150 (-300.2033, 130.4345) -> (-300.2033, 131.1433)
  spline S88 degree 2 poles (-300.2033, 131.1433) (-300.2033, 131.9291) (-301.5284, 131.9291) knots 0 0 0 1 1 1
  line L151 (-301.5284, 131.9291) -> (-302.7302, 131.9291)
  spline S89 degree 2 poles (-302.7302, 131.9291) (-304.4406, 131.9291) (-305.211, 132.5609) knots 0 0 0 1 1 1
  spline S90 degree 2 poles (-305.211, 132.5609) (-305.9814, 133.1926) (-305.9814, 134.4869) knots 0 0 0 1 1 1
  line L152 (-305.9814, 134.4869) -> (-305.9814, 135.1495)
  spline S91 degree 2 poles (-305.9814, 135.1495) (-305.9814, 136.9368) (-304.7025, 137.5686) knots 0 0 0 1 1 1
  spline S92 degree 2 poles (-304.7025, 137.5686) (-304.0862, 137.8921) (-303.3389, 138.0231) knots 0 0 0 1 1 1
  spline S93 degree 2 poles (-303.3389, 138.0231) (-302.5916, 138.1541) (-301.5438, 138.1541) knots 0 0 0 1 1 1
extrude "Extrude11" cut sketch "Sketch10" against normal blind 0.7 contours L6 L7 L8 L9 L10 L11 L12 L13 L14 L15 L16 L17 L18 L19 L20 L21 L22 L23 L24 L25 L26 L27 L28 L29 L30 L31 L32 L33 | L38 L39 L40 L41 L42 L43 L44 | L45 L46 L47 L48 L49 L50 L51 | L52 L53 L54 L55 L56 L57 L58 L59 L60 L61 L62 | S0 L66 L67 S1 L68 S2 S3 S4 S5 L69 S6 L70 L71 L72 S7 L73 S8 S9 S10 S11 L74 S12 S13 S14 L75 S15 S16 S17 L76 S18 S19 | L77 L78 L79 L80 | L81 L82 L83 L84 L85 L86 | L87 L88 L89 L90 L91 L92 L93 L94 L95 | L96 S20 S21 L97 S22 S23 L98 L99 L100 L101 L102 L103 L104 | S28 S29 S30 S31 L109 S32 S33 S34 S35 S36 S37 S38 S39 S40 S41 L110 S42 S43 S44 | L113 L114 L115 L116 L117 L118 | L119 L120 L121 L122 L123 L124 L125 L126 | L131 S57 S58 S59 L132 S60 S61 L133 S62 S63 L134 S64 S65 L135 L136 | S76 L145 S77 S78 L146 S79 S80 L147 S81 L148 S82 S83 S84 L149 S85 S86 S87 L150 S88 L151 S89 S90 L152 S91 S92 S93 bodies 4 5
extrude "Extrude12" add 22 faces at (0.7, 27.1447, -176.4134) (0.7, 38.108, -183.7699) (0.7, 43.5658, -194.726) (0.7, 21.6647, -282.6491) (0.7, 38.108, -283.7699) (0.7, 43.5658, -294.726) (0.7, 112.6739, -305.8966) (0.7, 113.1669, -288.7318) (0.7, 111.6415, -279.872) (0.7, 116.5568, -274.5664) (0.7, 111.6723, -269.1016) (0.7, 134.0966, -270.0954) (0.7, 133.2542, -284.9285) (0.7, 133.208, -289.325) (0.7, 136.7879, -299.1915) (0.7, 127.8636, -196.9158) (0.7, 119.9488, -170.9153) (0.7, 141.1342, -170.7513) (0.7, 136.7336, -179.6358) (0.7, 136.7336, -187.6789) (0.7, 135.5734, -196.4802) (0.7, 141.5965, -201.0795) along direction (-1, 0, 0) blind 0.7 separate body on bodies 1 3 4 5 makes body 6 at (0.7, 135.5734, -196.4802) makes body 7 at (0.7, 136.7336, -179.6358) makes body 8 at (0.7, 119.9488, -170.9153) makes body 9 at (0.7, 136.7879, -299.1915) makes body 10 at (0.7, 133.2542, -284.9285) makes body 11 at (0.7, 111.6723, -269.1016) makes body 12 at (0.7, 111.6415, -279.872) makes body 13 at (0.7, 112.6739, -305.8966) makes body 14 at (0.7, 38.108, -283.7699) makes body 15 at (0.7, 43.5658, -194.726) makes body 16 at (0.7, 27.1447, -176.4134) makes body 17 at (0.7, 38.108, -183.7699) makes body 18 at (0.7, 21.6647, -282.6491) makes body 19 at (0.7, 43.5658, -294.726) makes body 20 at (0.7, 113.1669, -288.7318) makes body 21 at (0.7, 116.5568, -274.5664) makes body 22 at (0.7, 134.0966, -270.0954) makes body 23 at (0.7, 133.208, -289.325) makes body 24 at (0.7, 127.8636, -196.9158) makes body 25 at (0.7, 141.1342, -170.7513) makes body 26 at (0.7, 136.7336, -187.6789) makes body 27 at (0.7, 141.5965, -201.0795)
move_body "Move5" bodies 4 8 25 26 24 16 15 17 7 3 27 6 to x (1, 0, 0) y (0, 1, 0) z (0, 0, 1) at (0, 0, -166)
move_body "Move6" bodies 5 27 6 4 24 26 10 20 23 9 12 11 13 22 8 21 7 25 to x (1, 0, 0) y (0, 1, 0) z (0, 0, 1) at (0, -150, 0)
move_body "Move7" bodies 2 to x (1, 0, 0) y (0, 0, 1) z (0, -1, 0) at (0, 163.3284, 149.6716)
sketch "Sketch11" plane through (0, 0, 0) normal (-1, 0, 0) x (0, 0, 1)
  line L0 (156.2929, 5.3284) -> (152.1716, 1.2071)
  line L1 (152.1716, 1.2071) -> (152.1716, -63.6716)
  line L2 (152.1716, -63.6716) -> (182.0503, -63.6716)
  line L3 (182.0503, -63.6716) -> (221.1716, -24.5503)
  line L4 (221.1716, -24.5503) -> (221.1716, 5.3284)
  line L5 (221.1716, 5.3284) -> (156.2929, 5.3284)
  line L6 (198.0219, -7.9451) -> (196.2191, -7.9458)
  line L7 (196.2191, -7.9458) -> (196.2167, -1.7285)
  line L8 (196.2167, -1.7285) -> (192.5303, -1.7299)
  line L9 (192.5303, -1.7299) -> (192.5298, -0.4472)
  line L10 (192.5298, -0.4472) -> (198.019, -0.4451)
  line L11 (198.019, -0.4451) -> (198.0219, -7.9451)
  line L12 (186.6737, -7.9494) -> (184.478, -7.9503)
  line L13 (184.478, -7.9503) -> (181.7709, -0.4513)
  line L14 (181.7709, -0.4513) -> (183.5968, -0.4506)
  line L15 (183.5968, -0.4506) -> (184.2678, -2.4265)
  line L16 (184.2678, -2.4265) -> (187.0067, -2.4254)
  line L17 (187.0067, -2.4254) -> (187.6646, -0.4491)
  line L18 (187.6646, -0.4491) -> (189.4443, -0.4484)
  line L19 (189.4443, -0.4484) -> (186.6737, -7.9494)
  line L20 (184.6612, -3.6282) -> (185.6099, -6.4475)
  line L21 (185.6099, -6.4475) -> (185.6561, -6.4475)
  line L22 (185.6561, -6.4475) -> (186.6027, -3.6274)
  line L23 (186.6027, -3.6274) -> (184.6612, -3.6282)
  line L24 (178.2838, -7.9527) -> (175.2446, -7.9539)
  spline S0 degree 2 poles (175.2446, -7.9539) (174.1698, -7.9543) (173.5862, -7.7985) knots 0 0 0 1 1 1
  spline S1 degree 2 poles (173.5862, -7.7985) (173.0025, -7.6427) (172.7597, -7.3019) knots 0 0 0 1 1 1
  spline S2 degree 2 poles (172.7597, -7.3019) (172.5169, -6.9611) (172.5167, -6.3486) knots 0 0 0 1 1 1
  line L25 (172.5167, -6.3486) -> (172.5163, -5.4241)
  spline S3 degree 2 poles (172.5163, -5.4241) (172.5162, -5.1121) (172.7645, -4.8346) knots 0 0 0 1 1 1
  spline S4 degree 2 poles (172.7645, -4.8346) (173.0129, -4.5572) (173.348, -4.4531) knots 0 0 0 1 1 1
  line L26 (173.348, -4.4531) -> (173.348, -4.3953)
  spline S5 degree 2 poles (173.348, -4.3953) (172.9088, -4.3492) (172.5447, -4.02) knots 0 0 0 1 1 1
  spline S6 degree 2 poles (172.5447, -4.02) (172.1805, -3.6908) (172.1803, -3.2863) knots 0 0 0 1 1 1
  line L27 (172.1803, -3.2863) -> (172.1799, -2.1307)
  spline S7 degree 2 poles (172.1799, -2.1307) (172.1796, -1.2178) (172.9074, -0.8361) knots 0 0 0 1 1 1
  spline S8 degree 2 poles (172.9074, -0.8361) (173.6353, -0.4545) (175.1608, -0.4539) knots 0 0 0 1 1 1
  line L28 (175.1608, -0.4539) -> (178.2809, -0.4527)
  line L29 (178.2809, -0.4527) -> (178.2838, -7.9527)
  spline S9 degree 2 poles (175.2434, -4.903) (174.8158, -4.9032) (174.6078, -4.9726) knots 0 0 0 1 1 1
  spline S10 degree 2 poles (174.6078, -4.9726) (174.3998, -5.042) (174.3248, -5.1981) knots 0 0 0 1 1 1
  spline S11 degree 2 poles (174.3248, -5.1981) (174.2497, -5.3541) (174.2498, -5.6546) knots 0 0 0 1 1 1
  line L30 (174.2498, -5.6546) -> (174.25, -6.0244)
  spline S12 degree 2 poles (174.25, -6.0244) (174.2501, -6.2901) (174.3195, -6.423) knots 0 0 0 1 1 1
  spline S13 degree 2 poles (174.3195, -6.423) (174.3889, -6.5559) (174.6027, -6.6136) knots 0 0 0 1 1 1
  spline S14 degree 2 poles (174.6027, -6.6136) (174.8165, -6.6713) (175.2787, -6.6711) knots 0 0 0 1 1 1
  line L31 (175.2787, -6.6711) -> (176.4806, -6.6706)
  line L32 (176.4806, -6.6706) -> (176.4799, -4.9025)
  line L33 (176.4799, -4.9025) -> (175.2434, -4.903)
  spline S15 degree 2 poles (175.1959, -1.7366) (174.5372, -1.7369) (174.2599, -1.8872) knots 0 0 0 1 1 1
  spline S16 degree 2 poles (174.2599, -1.8872) (173.9826, -2.0376) (173.9828, -2.3727) knots 0 0 0 1 1 1
  line L34 (173.9828, -2.3727) -> (173.983, -2.9736)
  spline S17 degree 2 poles (173.983, -2.9736) (173.9832, -3.3896) (174.197, -3.5629) knots 0 0 0 1 1 1
  spline S18 degree 2 poles (174.197, -3.5629) (174.4109, -3.7362) (174.954, -3.7359) knots 0 0 0 1 1 1
  line L35 (174.954, -3.7359) -> (176.4794, -3.7354)
  line L36 (176.4794, -3.7354) -> (176.4787, -1.7361)
  line L37 (176.4787, -1.7361) -> (175.1959, -1.7366)
  spline S19 degree 2 poles (165.858, -0.3419) (166.9327, -0.3415) (168.516, -0.5489) knots 0 0 0 1 1 1
  line L38 (168.516, -0.5489) -> (168.5165, -1.9241)
  spline S20 degree 2 poles (168.5165, -1.9241) (166.5518, -1.6244) (165.8353, -1.6247) knots 0 0 0 1 1 1
  spline S21 degree 2 poles (165.8353, -1.6247) (164.333, -1.6253) (164.3333, -2.3995) knots 0 0 0 1 1 1
  line L39 (164.3333, -2.3995) -> (164.3335, -2.8849)
  spline S22 degree 2 poles (164.3335, -2.8849) (164.3336, -3.2547) (164.5475, -3.4511) knots 0 0 0 1 1 1
  spline S23 degree 2 poles (164.5475, -3.4511) (164.7614, -3.6474) (165.3161, -3.6472) knots 0 0 0 1 1 1
  line L40 (165.3161, -3.6472) -> (166.1944, -3.6469)
  spline S24 degree 2 poles (166.1944, -3.6469) (168.6674, -3.6459) (168.6682, -5.6105) knots 0 0 0 1 1 1
  line L41 (168.6682, -5.6105) -> (168.6684, -6.1652)
  spline S25 degree 2 poles (168.6684, -6.1652) (168.6687, -7.1475) (167.8484, -7.61) knots 0 0 0 1 1 1
  spline S26 degree 2 poles (167.8484, -7.61) (167.0281, -8.0726) (165.2485, -8.0733) knots 0 0 0 1 1 1
  spline S27 degree 2 poles (165.2485, -8.0733) (164.324, -8.0736) (162.9025, -7.924) knots 0 0 0 1 1 1
  line L42 (162.9025, -7.924) -> (162.902, -6.5834)
  spline S28 degree 2 poles (162.902, -6.5834) (164.647, -6.7908) (165.3057, -6.7905) knots 0 0 0 1 1 1
  spline S29 degree 2 poles (165.3057, -6.7905) (166.2187, -6.7902) (166.5306, -6.6398) knots 0 0 0 1 1 1
  spline S30 degree 2 poles (166.5306, -6.6398) (166.8657, -6.4779) (166.8656, -6.1312) knots 0 0 0 1 1 1
  line L43 (166.8656, -6.1312) -> (166.8654, -5.5996)
  spline S31 degree 2 poles (166.8654, -5.5996) (166.8651, -5.0103) (165.8713, -5.0106) knots 0 0 0 1 1 1
  line L44 (165.8713, -5.0106) -> (164.9699, -5.011)
  spline S32 degree 2 poles (164.9699, -5.011) (163.6872, -5.0115) (163.1092, -4.5379) knots 0 0 0 1 1 1
  spline S33 degree 2 poles (163.1092, -4.5379) (162.5312, -4.0643) (162.5308, -3.0936) knots 0 0 0 1 1 1
  line L45 (162.5308, -3.0936) -> (162.5306, -2.5967)
  spline S34 degree 2 poles (162.5306, -2.5967) (162.5301, -1.2562) (163.4891, -0.782) knots 0 0 0 1 1 1
  spline S35 degree 2 poles (163.4891, -0.782) (163.9512, -0.5391) (164.5117, -0.4407) knots 0 0 0 1 1 1
  spline S36 degree 2 poles (164.5117, -0.4407) (165.0721, -0.3422) (165.858, -0.3419) knots 0 0 0 1 1 1
  line L46 (197.6342, -26.3322) -> (190.8855, -26.3783)
  spline S37 degree 2 poles (190.8855, -26.3783) (187.881, -26.3989) (186.5355, -25.68) knots 0 0 0 1 1 1
  spline S38 degree 2 poles (186.5355, -25.68) (185.19, -24.9611) (185.1784, -23.2508) knots 0 0 0 1 1 1
  line L47 (185.1784, -23.2508) -> (185.1604, -20.6161)
  spline S39 degree 2 poles (185.1604, -20.6161) (185.1514, -19.2987) (186.0823, -18.5412) knots 0 0 0 1 1 1
  spline S40 degree 2 poles (186.0823, -18.5412) (187.0132, -17.7836) (188.5603, -17.565) knots 0 0 0 1 1 1
  line L48 (188.5603, -17.565) -> (184.1731, -11.4238)
  line L49 (184.1731, -11.4238) -> (188.3332, -11.3954)
  line L50 (188.3332, -11.3954) -> (192.3025, -17.2621)
  line L51 (192.3025, -17.2621) -> (193.9666, -17.2508)
  line L52 (193.9666, -17.2508) -> (193.9263, -11.3572)
  line L53 (193.9263, -11.3572) -> (197.5318, -11.3326)
  line L54 (197.5318, -11.3326) -> (197.6342, -26.3322)
  spline S41 degree 2 poles (190.8858, -19.6524) (189.6147, -19.6611) (189.1547, -19.9994) knots 0 0 0 1 1 1
  spline S42 degree 2 poles (189.1547, -19.9994) (188.6948, -20.3377) (188.7014, -21.3084) knots 0 0 0 1 1 1
  line L55 (188.7014, -21.3084) -> (188.7087, -22.3715)
  spline S43 degree 2 poles (188.7087, -22.3715) (188.7143, -23.2036) (189.2134, -23.5122) knots 0 0 0 1 1 1
  spline S44 degree 2 poles (189.2134, -23.5122) (189.7124, -23.8208) (190.9142, -23.8126) knots 0 0 0 1 1 1
  line L56 (190.9142, -23.8126) -> (194.0112, -23.7914)
  line L57 (194.0112, -23.7914) -> (193.9828, -19.6313)
  line L58 (193.9828, -19.6313) -> (190.8858, -19.6524)
  spline S45 degree 2 poles (170.0039, -11.2895) (171.2519, -11.281) (172.3046, -11.4356) knots 0 0 0 1 1 1
  spline S46 degree 2 poles (172.3046, -11.4356) (173.3573, -11.5902) (174.4925, -11.9753) knots 0 0 0 1 1 1
  spline S47 degree 2 poles (174.4925, -11.9753) (175.7202, -12.383) (176.42, -13.3143) knots 0 0 0 1 1 1
  spline S48 degree 2 poles (176.42, -13.3143) (177.1197, -14.2456) (177.1289, -15.5861) knots 0 0 0 1 1 1
  line L59 (177.1289, -15.5861) -> (177.1737, -22.1499)
  spline S49 degree 2 poles (177.1737, -22.1499) (177.1813, -23.2592) (176.6904, -24.1409) knots 0 0 0 1 1 1
  spline S50 degree 2 poles (176.6904, -24.1409) (176.1995, -25.0225) (175.4172, -25.5364) knots 0 0 0 1 1 1
  spline S51 degree 2 poles (175.4172, -25.5364) (174.7268, -25.9802) (173.7119, -26.2876) knots 0 0 0 1 1 1
  spline S52 degree 2 poles (173.7119, -26.2876) (172.6971, -26.595) (171.8193, -26.6704) knots 0 0 0 1 1 1
  spline S53 degree 2 poles (171.8193, -26.6704) (171.0108, -26.7452) (170.1095, -26.7514) knots 0 0 0 1 1 1
  spline S54 degree 2 poles (170.1095, -26.7514) (169.0463, -26.7586) (168.26, -26.6831) knots 0 0 0 1 1 1
  spline S55 degree 2 poles (168.26, -26.6831) (167.4736, -26.6076) (166.5012, -26.36) knots 0 0 0 1 1 1
  spline S56 degree 2 poles (166.5012, -26.36) (165.3896, -26.044) (164.67, -25.5867) knots 0 0 0 1 1 1
  spline S57 degree 2 poles (164.67, -25.5867) (163.9503, -25.1293) (163.4593, -24.3006) knots 0 0 0 1 1 1
  spline S58 degree 2 poles (163.4593, -24.3006) (162.945, -23.4489) (162.9368, -22.2471) knots 0 0 0 1 1 1
  line L60 (162.9368, -22.2471) -> (162.8919, -15.6833)
  spline S59 degree 2 poles (162.8919, -15.6833) (162.8834, -14.4353) (163.536, -13.5294) knots 0 0 0 1 1 1
  spline S60 degree 2 poles (163.536, -13.5294) (164.1885, -12.6236) (165.3409, -12.1534) knots 0 0 0 1 1 1
  spline S61 degree 2 poles (165.3409, -12.1534) (167.4153, -11.3072) (170.0039, -11.2895) knots 0 0 0 1 1 1
  spline S62 degree 2 poles (169.9752, -13.8552) (169.2125, -13.8605) (168.6928, -13.9218) knots 0 0 0 1 1 1
  spline S63 degree 2 poles (168.6928, -13.9218) (168.1732, -13.9831) (167.6196, -14.1487) knots 0 0 0 1 1 1
  spline S64 degree 2 poles (167.6196, -14.1487) (167.0661, -14.3143) (166.7798, -14.6976) knots 0 0 0 1 1 1
  spline S65 degree 2 poles (166.7798, -14.6976) (166.4935, -15.0809) (166.4974, -15.6587) knots 0 0 0 1 1 1
  line L61 (166.4974, -15.6587) -> (166.5424, -22.2456)
  spline S66 degree 2 poles (166.5424, -22.2456) (166.5497, -23.3088) (167.4079, -23.7536) knots 0 0 0 1 1 1
  spline S67 degree 2 poles (167.4079, -23.7536) (168.2661, -24.1984) (170.0688, -24.1861) knots 0 0 0 1 1 1
  spline S68 degree 2 poles (170.0688, -24.1861) (171.8716, -24.1738) (172.7237, -23.7288) knots 0 0 0 1 1 1
  spline S69 degree 2 poles (172.7237, -23.7288) (173.5759, -23.2839) (173.5684, -22.1976) knots 0 0 0 1 1 1
  line L62 (173.5684, -22.1976) -> (173.5234, -15.6107)
  spline S70 degree 2 poles (173.5234, -15.6107) (173.5195, -15.0329) (173.2164, -14.6536) knots 0 0 0 1 1 1
  spline S71 degree 2 poles (173.2164, -14.6536) (172.9134, -14.2743) (172.3345, -14.1165) knots 0 0 0 1 1 1
  spline S72 degree 2 poles (172.3345, -14.1165) (171.7787, -13.9585) (171.2583, -13.9043) knots 0 0 0 1 1 1
  spline S73 degree 2 poles (171.2583, -13.9043) (170.7379, -13.85) (169.9752, -13.8552) knots 0 0 0 1 1 1
  line L63 (197.1975, -44.6519) -> (193.5921, -44.6187)
  line L64 (193.5921, -44.6187) -> (193.73, -29.6194)
  line L65 (193.73, -29.6194) -> (197.3354, -29.6525)
  line L66 (197.3354, -29.6525) -> (197.1975, -44.6519)
  line L67 (193.5645, -37.5689) -> (187.8836, -44.5663)
  line L68 (187.8836, -44.5663) -> (183.6542, -44.5274)
  line L69 (183.6542, -44.5274) -> (189.4038, -37.6)
  line L70 (189.4038, -37.6) -> (183.168, -29.5223)
  line L71 (183.168, -29.5223) -> (187.5592, -29.5626)
  line L72 (187.5592, -29.5626) -> (193.5645, -37.5689)
  line L73 (172.2042, -35.431) -> (177.5527, -44.4713)
  line L74 (177.5527, -44.4713) -> (173.462, -44.4337)
  line L75 (173.462, -44.4337) -> (170.3497, -38.5343)
  line L76 (170.3497, -38.5343) -> (167.1526, -44.3758)
  line L77 (167.1526, -44.3758) -> (163.0387, -44.338)
  line L78 (163.0387, -44.338) -> (168.5983, -35.4441)
  line L79 (168.5983, -35.4441) -> (168.654, -29.3889)
  line L80 (168.654, -29.3889) -> (172.2594, -29.4221)
  line L81 (172.2594, -29.4221) -> (172.2042, -35.431)
extrude "Extrude13" cut sketch "Sketch11" against normal blind 0.7 contours L6 L7 L8 L9 L10 L11 | L12 L13 L14 L15 L16 L17 L18 L19 | L24 S0 S1 S2 L25 S3 S4 L26 S5 S6 L27 S7 S8 L28 L29 | S19 L38 S20 S21 L39 S22 S23 L40 S24 L41 S25 S26 S27 L42 S28 S29 S30 L43 S31 L44 S32 S33 L45 S34 S35 S36 | L46 S37 S38 L47 S39 S40 L48 L49 L50 L51 L52 L53 L54 | S45 S46 S47 S48 L59 S49 S50 S51 S52 S53 S54 S55 S56 S57 S58 L60 S59 S60 S61 | L63 L64 L65 L66 | L67 L68 L69 L70 L71 L72 | L73 L74 L75 L76 L77 L78 L79 L80 L81 bodies 2
move_body "Move8" bodies 11 23 9 5 10 13 20 12 21 22 to x (1, 0, 0) y (0, 1, 0) z (0, 0, 1) at (0, 0, 150)
move_body "Move9" bodies 2 to x (1, 0, 0) y (0, 1, 0) z (0, 0, 1) at (0, -7.6815, -469.9971)
extrude "Extrude14" add 9 faces at (0.7, -11.0544, -272.5779) (0.7, -42.3227, -273.9094) (0.7, -26.7802, -273.6141) (0.7, -39.9098, -283.2867) (0.7, -47.1604, -296.6282) (0.7, -27.732, -304.6715) (0.7, -11.6915, -286.3604) (0.7, -11.7284, -292.3157) (0.7, -9.0474, -302.3745) along direction (-1, 0, 0) blind 0.7 separate body on bodies 2 makes body 28 at (0.7, -11.7284, -292.3157) makes body 29 at (0.7, -27.732, -304.6715) makes body 30 at (0.7, -39.9098, -283.2867) makes body 31 at (0.7, -42.3227, -273.9094) makes body 32 at (0.7, -11.0544, -272.5779) makes body 33 at (0.7, -26.7802, -273.6141) makes body 34 at (0.7, -47.1604, -296.6282) makes body 35 at (0.7, -11.6915, -286.3604) makes body 36 at (0.7, -9.0474, -302.3745)
delete_face "DeleteFace2" 1 faces at (21.5, -49.5602, -318.3255) on bodies 2
delete_face "DeleteFace3" 1 faces at (21.5, 49.7071, -317.5) on bodies 1
delete_face "DeleteFace4" 1 faces at (21.4251, -2.881, -315.0451) on bodies 2
delete_face "DeleteFace5" 1 faces at (21.5, 5.3452, -316.431) on bodies 1
delete_face "DeleteFace6" 1 faces at (15.0255, -71.4966, -319.2192) on bodies 2
delete_face "DeleteFace7" 1 faces at (15.1364, -6.0544, -319.2246) on bodies 2
delete_face "DeleteFace8" 1 faces at (14.2722, -1.0628, -314.3887) on bodies 2
delete_face "DeleteFace9" 1 faces at (14.2752, 1.2144, -313.5725) on bodies 1
delete_face "DeleteFace10" 1 faces at (15.1364, 5.929, -318.2864) on bodies 1
chamfer "Chamfer16" distance 5 angle 45 1 edges at (22, -38.6031, -319.3255) on bodies 2
delete_face "DeleteFace11" 1 faces at (14.7187, 72.0291, -318.2149) on bodies 1
chamfer "Chamfer17" distance 5 angle 45 1 edges at (22, 38.75, -318.5) on bodies 1
fillet "Fillet6" radius 2 2 edges at (9.25, 73, -318.5) (9.25, -72.8531, -319.3255) on bodies 1 2
chamfer "Chamfer18" distance 1 angle 45 4 edges at (17, 38.5, -318.5) (17.5858, 72.4142, -317.9142) (19.75, 73, -315.75) (19.125, 3.875, -316.375) on bodies 1
chamfer "Chamfer19" distance 1 angle 45 4 edges at (19.125, -3.7281, -317.2005) (17, -38.3531, -319.3255) (19.75, -72.8531, -316.5755) (17.5858, -72.2673, -318.7397) on bodies 2
fillet "Fillet7" radius 1 4 edges at (8.6376, 6, -318.5) (11, 1, -313.5) (11, -0.8531, -314.3255) (8.6376, -5.8531, -319.3255) on bodies 1 2
